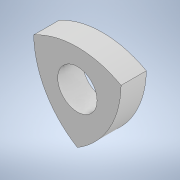
# Autodesk Inventor part: Rotor_test
Saved by Autodesk Inventor 2021 (Build 250183000, 183)
## iProperties
Created: 2021-03-22
Part Number: Rotor_test
Material: Generic
Document SubType Name: Modeling
Designer: lucia
Density: 1 g/cm^3
Appearance: Default
Author: lucia
Autodesk Inventor part; units mm, degrees
ref_plane "YZ Plane" through (0, 0, 0) normal (1, 0, 0) x (0, 1, 0)
ref_plane "XZ Plane" through (0, 0, 0) normal (0, 1, 0) x (-1, 0, 0)
ref_plane "XY Plane" through (0, 0, 0) normal (0, 0, 1) x (1, 0, 0)
sketch "Sketch1" plane through (0, 0, 0) normal (0, 0, 1) x (1, 0, 0)
  line L0 (0, -50.8) -> (-43.9941, 25.4)
  line L1 (43.9941, 25.4) -> (0, -50.8)
  line L2 (-43.9941, 25.4) -> (43.9941, 25.4)
  line L3 (0, -50.8) -> (0, 0)
  line L4 (0, 0) -> (41.6526, 0)
  line L5 (0, 37.592) -> (0, 36.7982)
  arc A0 (43.9941, 25.4) -> (-43.9941, 25.4) centre (0, -53.8034) ccw
  arc A1 (0, -50.8) -> (43.9941, 25.4) centre (-46.5951, 26.9017) ccw
  arc A2 (-43.9941, 25.4) -> (0, -50.8) centre (46.5951, 26.9017) ccw
  circle A3 centre (0, 0) radius 19.812
  point P0 (57.404, -6.604)
  dimension "d7" = 30
  dimension "d8" = 30
  dimension "d9" = 0.7937
  dimension "d10" = 39.624
  constraints: 12 end point, 7 point on circle, 4 centre point, 2 equal radius, 2 vertical, 1 coincident, 1 perpendicular, 8 other
  measures "d7" angle of L3 L1
  measures "d8" angle of L3 L0
  measures "d9" distance of L5.start L5.end
  measures "d10" diameter of A3
extrude "Extrusion1" add sketch "Sketch1" along normal blind 25.4 contours A2 L0 | L3 A3 L4 L1 | L0 L2 L1 L4 A3 L3 | L1 L4 A1 | A0 L2 | L1 A1 L4
body "Solid1"
